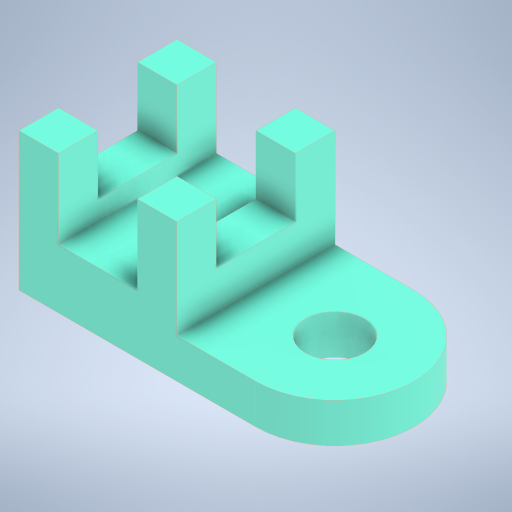
# Autodesk Inventor part: ASN4-TUT-BK
Saved by Autodesk Inventor 2024 (Build 280153000, 153)
## iProperties
Created: 2023-09-23
Part Number: ASN4-TUT-BK
Material: Copper, Cast
Document SubType Name: Modeling
Designer: bennk
Density: 8.94 g/cm^3
Appearance: Copper - Satin
Author: bennk
Autodesk Inventor part; units mm, degrees
ref_plane "YZ Plane" through (0, 0, 0) normal (1, 0, 0) x (0, 1, 0)
ref_plane "XZ Plane" through (0, 0, 0) normal (0, 1, 0) x (-1, 0, 0)
ref_plane "XY Plane" through (0, 0, 0) normal (0, 0, 1) x (1, 0, 0)
sketch "SIDE PROFILE" plane through (0, 0, 0) normal (0, 0, 1) x (1, 0, 0)
  line L0 (-38.1, 0) -> (38.1, 0)
  line L1 (-38.1, 0) -> (-38.1, 44.45)
  line L2 (-38.1, 44.45) -> (-25.4, 44.45)
  line L3 (-25.4, 44.45) -> (-25.4, 19.05)
  line L4 (-25.4, 19.05) -> (0, 19.05)
  line L5 (0, 19.05) -> (0, 44.45)
  line L6 (0, 44.45) -> (12.7, 44.45)
  line L7 (12.7, 44.45) -> (12.7, 12.7)
  line L8 (38.1, 0) -> (38.1, 12.7)
  line L9 (38.1, 12.7) -> (12.7, 12.7)
  point P0 (0, 0)
  dimension "d0" = 76.2
  dimension "d1" = 38.1
  dimension "d2" = 44.45
  dimension "d3" = 12.7
  dimension "d4" = 25.4
  dimension "d5" = 25.4
  dimension "d6" = 25.4
  dimension "d7" = 12.7
  dimension "d8" = 31.75
  dimension "d21" = 25.4
  dimension "d22" = 38.1
  constraints: 20 end point, 5 perpendicular, 3 vertical, 2 horizontal
  measures "d0" distance of L0.start L0.end
  measures "d1" distance of L0.start point (0, 0)
  measures "d2" distance of L0.start L1.end
  measures "d3" distance of L1.end L2.end
  measures "d4" distance of L2.end L3.end
  measures "d5" distance of L3.end L4.end
  measures "d6" distance of L4.end L5.end
  measures "d7" distance of L5.end L6.end
  measures "d8" distance of L6.end L7.end
  measures "d21" distance of L8.end L7.end
  measures "d22" distance from line of point (0, 0) L8
extrude "SIDE PROFILE EXTRUSION" add sketch "SIDE PROFILE" along normal blind 50.8
sketch "SEMICIRCLE" plane through (12.7, 12.7, 0) normal (0, 1, 0) x (1, 0, 0)
  line L0 (25.4, 0) -> (25.4, -50.8) projected
  line L1 (25.4, -50.8) -> (0, -50.8) projected
  circle A0 centre (25.4, -25.4) radius 25.4
  point P0 (-12.7, 0)
  constraints: 1 midpoint, 1 vertical alignment, 2 other
extrude "FRONT ROUNDING" add sketch "SEMICIRCLE" against normal blind 12.7
sketch "CIRCLE" plane through (12.7, 12.7, 50.8) normal (0, 1, 0) x (1, 0, 0)
  arc A0 (25.4, 0) -> (25.4, 50.8) centre (25.4, 25.4) ccw projected
  circle A1 centre (25.4, 25.4) radius 9.525
  point P0 (-12.7, 50.8)
  dimension "d13" = 19.05
  constraints: 1 centre point, 1 coincident
  measures "d13" diameter of A1
extrude "HOLE CUTOUT" cut sketch "CIRCLE" against normal blind 12.7
sketch "RECTANGLE" plane through (12.7, 12.7, 0) normal (1, 0, 0) x (0, 0, -1)
  line L0 (0, 31.75) -> (-50.8, 31.75) projected
  line L1 (-38.1, 31.75) -> (-12.7, 31.75)
  line L2 (-12.7, 31.75) -> (-12.7, 12.7)
  line L3 (-12.7, 12.7) -> (-38.1, 12.7)
  line L4 (-38.1, 12.7) -> (-38.1, 31.75)
  line L5 (0, 0) -> (0, 31.75) projected
  point P0 (0, -12.7)
  point P1 (-25.4, 31.75)
  dimension "d16" = 25.4
  dimension "d17" = 19.05
  dimension "d18" = 12.7
  constraints: 8 end point, 2 parallel, 1 horizontal, 1 midpoint, 1 perpendicular, 1 point on line
  measures "d16" distance of L2.end L3.end
  measures "d17" distance from line of point (-25.4, 31.75) L3
  measures "d18" distance between parallel lines of L5 L2
extrude "RECTANGULAR CUTOUT" cut sketch "RECTANGLE" against normal through all
body "Solid1"
